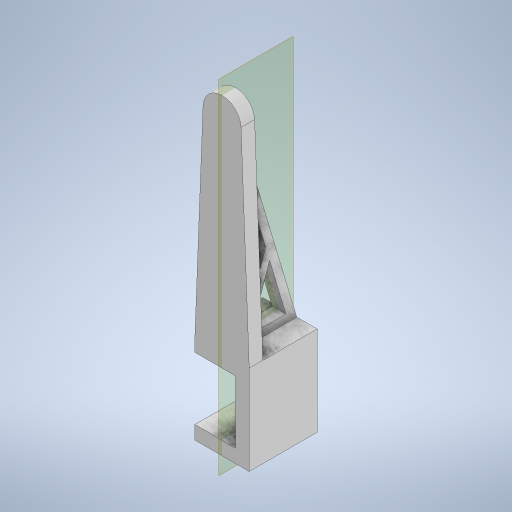
# Autodesk Inventor part: 전체 형상
Saved by Autodesk Inventor 2023 (Build 270158000, 158)
## iProperties
Created: 2022-11-11
Part Number: 전체 형상
Material: 일반
Document SubType Name: Modeling
Designer: hyunsu
Density: 1 g/cm^3
Appearance: 기본값
Author: hyunsu
Autodesk Inventor part; units mm, degrees
ref_plane "YZ Plane" through (0, 0, 0) normal (1, 0, 0) x (0, 1, 0)
ref_plane "XZ Plane" through (0, 0, 0) normal (0, 1, 0) x (-1, 0, 0)
ref_plane "XY Plane" through (0, 0, 0) normal (0, 0, 1) x (1, 0, 0)
sketch "스케치1" plane through (0, 0, 0) normal (0, 0, 1) x (1, 0, 0)
  line L0 (-5, -33) -> (5, -33)
  line L1 (5, -33) -> (5, 33)
  line L2 (5, 33) -> (-5, 33)
  line L3 (-5, 33) -> (-5, -33)
  line L4 (-5, -33) -> (5, 33) construction
  line L5 (5, -33) -> (-5, 33) construction
  line L6 (-5, 33) -> (-35, 33)
  line L7 (-35, 33) -> (-35, 23)
  line L8 (-35, 23) -> (-5, 23)
  line L9 (-5, 23) -> (-5, 33)
  line L10 (0, 0) -> (-11.0402, 0)
  line L11 (-5, -33) -> (-35, -33)
  line L12 (-35, -33) -> (-35, -23)
  line L13 (-35, -23) -> (-5, -23)
  point P0 (-5, 23)
  point P1 (-5, -23)
  dimension "d0" = 66
  dimension "d1" = 10
  dimension "d2" = 10
  dimension "d3" = 30
  constraints: 28 end point, 4 parallel, 3 horizontal, 3 symmetric about line, 2 midpoint, 2 perpendicular
  measures "d0" distance of L0.end L1.end
  measures "d1" distance of L1.end L2.end
  measures "d2" distance of L6.end L7.end
  measures "d3" distance of L2.end L6.end
extrude "돌출1" add sketch "스케치1" along normal mid plane 50
sketch "스케치2" plane through (0, 0, 25) normal (0, 0, 1) x (1, 0, 0)
  circle A0 centre (-15, 183) radius 14
  line L0 (-35, 33) -> (-35, 23) projected
  line L1 (-35, 33) -> (-28.9889, 183.5585)
  line L2 (5, 33) -> (-35, 33) projected
  line L3 (-15, 33) -> (-15, 183) construction
  line L4 (5, 33) -> (-1.0111, 183.5585)
  point P0 (0, 0)
  dimension "d6" = 28
  dimension "d7" = 150
  constraints: 6 end point, 1 coincident, 1 midpoint, 1 symmetric about line, 1 vertical, 4 other
  measures "d7" distance of L3.start L3.end
extrude "돌출2" add sketch "스케치2" against normal blind 10
ref_plane "작업 평면1" through (-15, 23, -25) normal (-1, 0, 0) x (0, 0, 1)
sketch "스케치3" plane through (-15, 23, -25) normal (-1, 0, 0) x (0, 0, 1)
  line L0 (40, 160.5585) -> (40, 10) projected
  line L1 (0, 10) -> (40, 10) projected
  line L2 (40, 144.5585) -> (0, 10)
  line L3 (45.7513, 142.8488) -> (8.0431, 16)
  line L4 (8.0431, 16) -> (34, 16)
  line L5 (34, 16) -> (34, 160.5585)
  line L6 (34, 16) -> (20, 56.2226)
  line L7 (34, 34.2526) -> (22.9265, 66.0672)
  point P0 (25, -23)
  point P1 (34, 103.318)
  point P2 (34, 124.3747)
  point P3 (40, 123.5018)
  dimension "d10" = 16
  dimension "d11" = 6
  dimension "d12" = 6
  constraints: 12 end point, 4 point on line, 1 parallel, 2 other
  measures "d10" distance of L0.start L2.start
  measures "d11" distance between parallel lines of L2 L3
  measures "d12" distance between parallel lines of L6 L7
extrude "돌출3" add sketch "스케치3" along normal mid plane 10 contours L0 L3 L5 L2 | L0 L1 L2 L5 L3 | L7 L5 L6 L3
